Autodesk Inventor part; units mm, degrees
(part 4 of 4)
  line L1289 (-18.1511, -3.5265) -> (-17.9502, -3.8747) construction
  line L1290 (-17.9502, -3.8747) -> (-17.7035, -4.3021) construction
  line L1291 (-17.7035, -4.3021) -> (-17.3591, -4.6088) construction
  line L1292 (-17.3591, -4.6088) -> (-16.8809, -4.76) construction
  line L1293 (-16.8809, -4.76) -> (-16.5137, -4.8761) construction
  line L1294 (-16.5137, -4.8761) -> (-16.1388, -4.8972) construction
  line L1295 (-16.1388, -4.8972) -> (-15.7609, -4.8632) construction
  line L1296 (-15.7609, -4.8632) -> (-15.344, -4.8257) construction
  line L1297 (-15.344, -4.8257) -> (-14.9284, -4.7723) construction
  line L1298 (-14.9284, -4.7723) -> (-14.5126, -4.7225) construction
  line L1299 (-14.5126, -4.7225) -> (-14.3097, -4.6982) construction
  line L1300 (-14.3097, -4.6982) -> (-14.1058, -4.6758) construction
  line L1301 (-14.1058, -4.6758) -> (-13.906, -4.6349) construction
  line L1302 (-13.906, -4.6349) -> (-13.7036, -4.5936) construction
  line L1303 (-13.7036, -4.5936) -> (-13.5886, -4.433) construction
  line L1304 (-13.5886, -4.433) -> (-13.6065, -4.2455) construction
  line L1305 (-13.6065, -4.2455) -> (-13.6174, -4.1315) construction
  line L1306 (-13.6174, -4.1315) -> (-13.6744, -4.0385) construction
  line L1307 (-13.6744, -4.0385) -> (-13.7549, -3.96) construction
  line L1308 (-13.7549, -3.96) -> (-13.9237, -3.7955) construction
  line L1309 (-13.9237, -3.7955) -> (-14.1348, -3.7365) construction
  line L1310 (-14.1348, -3.7365) -> (-14.3597, -3.76) construction
  line L1311 (-14.3597, -3.76) -> (-14.6956, -3.7951) construction
  line L1312 (-14.6956, -3.7951) -> (-15.0291, -3.8532) construction
  line L1313 (-15.0291, -3.8532) -> (-15.364, -3.8988) construction
  line L1314 (-15.364, -3.8988) -> (-15.6048, -3.9316) construction
  line L1315 (-15.6048, -3.9316) -> (-15.8454, -3.9714) construction
  line L1316 (-15.8454, -3.9714) -> (-16.0874, -3.9874) construction
  line L1317 (-16.0874, -3.9874) -> (-16.4238, -4.0097) construction
  line L1318 (-16.4238, -4.0097) -> (-16.7238, -3.9011) construction
  line L1319 (-16.7238, -3.9011) -> (-16.9435, -3.6427) construction
  line L1320 (-16.9435, -3.6427) -> (-17.3408, -3.1754) construction
  line L1321 (-17.3408, -3.1754) -> (-17.5623, -2.6346) construction
  line L1322 (-17.5623, -2.6346) -> (-17.5206, -2.0131) construction
  line L1323 (-17.5206, -2.0131) -> (-17.4887, -1.5389) construction
  line L1324 (-17.4887, -1.5389) -> (-17.2384, -1.2172) construction
  line L1325 (-17.2384, -1.2172) -> (-16.7786, -1.0684) construction
  line L1326 (-16.7786, -1.0684) -> (-16.3846, -0.9409) construction
  line L1327 (-16.3846, -0.9409) -> (-15.9768, -0.89) construction
  line L1328 (-15.9768, -0.89) -> (-15.5673, -0.8506) construction
  line L1329 (-15.5673, -0.8506) -> (-15.3662, -0.8312) construction
  line L1330 (-15.3662, -0.8312) -> (-15.164, -0.8225) construction
  line L1331 (-15.164, -0.8225) -> (-14.9622, -0.8103) construction
  line L1332 (-14.9622, -0.8103) -> (-14.8743, -0.805) construction
  line L1333 (-14.8743, -0.805) -> (-14.7969, -0.7758) construction
  line L1334 (-14.7969, -0.7758) -> (-14.7522, -0.6983) construction
  line L1335 (-14.7522, -0.6983) -> (-14.6073, -0.4469) construction
  line L1336 (-14.6073, -0.4469) -> (-14.6652, -0.192) construction
  line L1337 (-14.6652, -0.192) -> (-14.9177, -0.0574) construction
  line L1338 (-14.9177, -0.0574) -> (-15.0775, 0.0278) construction
  line L1339 (-15.0775, 0.0278) -> (-15.2502, 0.0492) construction
  line L1340 (-15.2502, 0.0492) -> (-15.4261, 0.0563) construction
  line L1341 (-15.4261, 0.0563) -> (-15.7781, 0.0704) construction
  line L1342 (-15.7781, 0.0704) -> (-16.1265, 0.0344) construction
  line L1343 (-16.1265, 0.0344) -> (-16.473, -0.026) construction
  line L1344 (-16.473, -0.026) -> (-16.8039, -0.0836) construction
  line L1345 (-16.8039, -0.0836) -> (-17.133, -0.1458) construction
  line L1346 (-17.133, -0.1458) -> (-17.439, -0.2941) construction
  line L1347 (-17.439, -0.2941) -> (-17.8084, -0.4732) construction
  line L1348 (-17.8084, -0.4732) -> (-18.0982, -0.7312) construction
  line L1349 (-18.0982, -0.7312) -> (-18.265, -1.1138) construction
  line L1350 (-18.265, -1.1138) -> (-18.3824, -1.3828) construction
  line L1351 (-18.3824, -1.3828) -> (-18.4168, -1.6658) construction
  line L1352 (-18.4168, -1.6658) -> (-18.4071, -1.9562) construction
  spline S14 degree 3 poles (-36.9183, 1.2424) (-36.6709, 1.199) (-36.4382, 1.1494) (-36.203, 1.1193) (-35.8877, 1.079) (-35.57, 1.0809) (-35.2581, 1.146) (-35.1542, 1.1676) (-35.0599, 1.235) (-34.9579, 1.283) (-34.9598, 1.2682) (-34.9615, 1.2412) (-34.9669, 1.215) (-35.0299, 0.9055) (-35.0965, 0.5966) (-35.1557, 0.2864) (-35.1823, 0.1473) (-35.1758, 0.1419) (-35.3193, 0.1406) (-35.6164, 0.138) (-35.9136, 0.1414) (-36.2107, 0.1399) (-36.3909, 0.139) (-36.5712, 0.1357) (-36.7512, 0.1286) (-36.8096, 0.1264) (-36.8273, 0.1474) (-36.8315, 0.2021) (-36.855, 0.5079) (-36.8811, 0.8134) (-36.9065, 1.1191) (-36.91, 1.1614) (-36.9146, 1.2037) (-36.9183, 1.2424) knots 0 0 0 0 1 1 1 2 2 2 3 3 3 4 4 4 5 5 5 6 6 6 7 7 7 8 8 8 9 9 9 10 10 10 11 11 11 11
  line L1353 (-36.9183, 1.2424) -> (-36.6709, 1.199) construction
  line L1354 (-36.6709, 1.199) -> (-36.4382, 1.1494) construction
  line L1355 (-36.4382, 1.1494) -> (-36.203, 1.1193) construction
  line L1356 (-36.203, 1.1193) -> (-35.8877, 1.079) construction
  line L1357 (-35.8877, 1.079) -> (-35.57, 1.0809) construction
  line L1358 (-35.57, 1.0809) -> (-35.2581, 1.146) construction
  line L1359 (-35.2581, 1.146) -> (-35.1542, 1.1676) construction
  line L1360 (-35.1542, 1.1676) -> (-35.0599, 1.235) construction
  line L1361 (-35.0599, 1.235) -> (-34.9579, 1.283) construction
  line L1362 (-34.9579, 1.283) -> (-34.9598, 1.2682) construction
  line L1363 (-34.9598, 1.2682) -> (-34.9615, 1.2412) construction
  line L1364 (-34.9615, 1.2412) -> (-34.9669, 1.215) construction
  line L1365 (-34.9669, 1.215) -> (-35.0299, 0.9055) construction
  line L1366 (-35.0299, 0.9055) -> (-35.0965, 0.5966) construction
  line L1367 (-35.0965, 0.5966) -> (-35.1557, 0.2864) construction
  line L1368 (-35.1557, 0.2864) -> (-35.1823, 0.1473) construction
  line L1369 (-35.1823, 0.1473) -> (-35.1758, 0.1419) construction
  line L1370 (-35.1758, 0.1419) -> (-35.3193, 0.1406) construction
  line L1371 (-35.3193, 0.1406) -> (-35.6164, 0.138) construction
  line L1372 (-35.6164, 0.138) -> (-35.9136, 0.1414) construction
  line L1373 (-35.9136, 0.1414) -> (-36.2107, 0.1399) construction
  line L1374 (-36.2107, 0.1399) -> (-36.3909, 0.139) construction
  line L1375 (-36.3909, 0.139) -> (-36.5712, 0.1357) construction
  line L1376 (-36.5712, 0.1357) -> (-36.7512, 0.1286) construction
  line L1377 (-36.7512, 0.1286) -> (-36.8096, 0.1264) construction
  line L1378 (-36.8096, 0.1264) -> (-36.8273, 0.1474) construction
  line L1379 (-36.8273, 0.1474) -> (-36.8315, 0.2021) construction
  line L1380 (-36.8315, 0.2021) -> (-36.855, 0.5079) construction
  line L1381 (-36.855, 0.5079) -> (-36.8811, 0.8134) construction
  line L1382 (-36.8811, 0.8134) -> (-36.9065, 1.1191) construction
  line L1383 (-36.9065, 1.1191) -> (-36.91, 1.1614) construction
  line L1384 (-36.91, 1.1614) -> (-36.9146, 1.2037) construction
  line L1385 (-36.9146, 1.2037) -> (-36.9183, 1.2424) construction
  spline S15 degree 3 poles (-30.21, 0.1155) (-30.4884, 0.1155) (-30.749, 0.1155) (-31.0096, 0.1155) (-31.0949, 0.1155) (-31.1802, 0.1169) (-31.2655, 0.1151) (-31.3106, 0.1141) (-31.3296, 0.129) (-31.3324, 0.1776) (-31.3492, 0.4716) (-31.3731, 0.7652) (-31.386, 1.0594) (-31.3905, 1.1624) (-31.3737, 1.2669) (-31.3602, 1.3699) (-31.3526, 1.4281) (-31.3153, 1.4376) (-31.2641, 1.4089) (-31.105, 1.3198) (-30.9887, 1.1846) (-30.8818, 1.0429) (-30.6662, 0.7573) (-30.4571, 0.4669) (-30.2457, 0.1781) (-30.235, 0.1635) (-30.2276, 0.1466) (-30.21, 0.1155) knots 0 0 0 0 1 1 1 2 2 2 3 3 3 4 4 4 5 5 5 6 6 6 7 7 7 8 8 8 9 9 9 9
  line L1386 (-30.21, 0.1155) -> (-30.4884, 0.1155) construction
  line L1387 (-30.4884, 0.1155) -> (-30.749, 0.1155) construction
  line L1388 (-30.749, 0.1155) -> (-31.0096, 0.1155) construction
  line L1389 (-31.0096, 0.1155) -> (-31.0949, 0.1155) construction
  line L1390 (-31.0949, 0.1155) -> (-31.1802, 0.1169) construction
  line L1391 (-31.1802, 0.1169) -> (-31.2655, 0.1151) construction
  line L1392 (-31.2655, 0.1151) -> (-31.3106, 0.1141) construction
  line L1393 (-31.3106, 0.1141) -> (-31.3296, 0.129) construction
  line L1394 (-31.3296, 0.129) -> (-31.3324, 0.1776) construction
  line L1395 (-31.3324, 0.1776) -> (-31.3492, 0.4716) construction
  line L1396 (-31.3492, 0.4716) -> (-31.3731, 0.7652) construction
  line L1397 (-31.3731, 0.7652) -> (-31.386, 1.0594) construction
  line L1398 (-31.386, 1.0594) -> (-31.3905, 1.1624) construction
  line L1399 (-31.3905, 1.1624) -> (-31.3737, 1.2669) construction
  line L1400 (-31.3737, 1.2669) -> (-31.3602, 1.3699) construction
  line L1401 (-31.3602, 1.3699) -> (-31.3526, 1.4281) construction
  line L1402 (-31.3526, 1.4281) -> (-31.3153, 1.4376) construction
  line L1403 (-31.3153, 1.4376) -> (-31.2641, 1.4089) construction
  line L1404 (-31.2641, 1.4089) -> (-31.105, 1.3198) construction
  line L1405 (-31.105, 1.3198) -> (-30.9887, 1.1846) construction
  line L1406 (-30.9887, 1.1846) -> (-30.8818, 1.0429) construction
  line L1407 (-30.8818, 1.0429) -> (-30.6662, 0.7573) construction
  line L1408 (-30.6662, 0.7573) -> (-30.4571, 0.4669) construction
  line L1409 (-30.4571, 0.4669) -> (-30.2457, 0.1781) construction
  line L1410 (-30.2457, 0.1781) -> (-30.235, 0.1635) construction
  line L1411 (-30.235, 0.1635) -> (-30.2276, 0.1466) construction
  line L1412 (-30.2276, 0.1466) -> (-30.21, 0.1155) construction
  spline S16 degree 3 poles (-33.0561, 0.1374) (-33.4981, 0.1374) (-33.9277, 0.1374) (-34.3711, 0.1374) (-34.3433, 0.2083) (-34.3243, 0.2629) (-34.3009, 0.3155) (-34.2271, 0.4812) (-34.1924, 0.6625) (-34.0848, 0.8154) (-33.9271, 1.0395) (-33.6943, 1.0697) (-33.5072, 0.8689) (-33.4206, 0.7759) (-33.3543, 0.6625) (-33.2866, 0.5536) (-33.2162, 0.4401) (-33.155, 0.3209) (-33.0901, 0.2041) (-33.0787, 0.1836) (-33.0687, 0.1623) (-33.0561, 0.1374) knots 0 0 0 0 1 1 1 2 2 2 3 3 3 4 4 4 5 5 5 6 6 6 7 7 7 7
  line L1413 (-33.0561, 0.1374) -> (-33.4981, 0.1374) construction
  line L1414 (-33.4981, 0.1374) -> (-33.9277, 0.1374) construction
  line L1415 (-33.9277, 0.1374) -> (-34.3711, 0.1374) construction
  line L1416 (-34.3711, 0.1374) -> (-34.3433, 0.2083) construction
  line L1417 (-34.3433, 0.2083) -> (-34.3243, 0.2629) construction
  line L1418 (-34.3243, 0.2629) -> (-34.3009, 0.3155) construction
  line L1419 (-34.3009, 0.3155) -> (-34.2271, 0.4812) construction
  line L1420 (-34.2271, 0.4812) -> (-34.1924, 0.6625) construction
  line L1421 (-34.1924, 0.6625) -> (-34.0848, 0.8154) construction
  line L1422 (-34.0848, 0.8154) -> (-33.9271, 1.0395) construction
  line L1423 (-33.9271, 1.0395) -> (-33.6943, 1.0697) construction
  line L1424 (-33.6943, 1.0697) -> (-33.5072, 0.8689) construction
  line L1425 (-33.5072, 0.8689) -> (-33.4206, 0.7759) construction
  line L1426 (-33.4206, 0.7759) -> (-33.3543, 0.6625) construction
  line L1427 (-33.3543, 0.6625) -> (-33.2866, 0.5536) construction
  line L1428 (-33.2866, 0.5536) -> (-33.2162, 0.4401) construction
  line L1429 (-33.2162, 0.4401) -> (-33.155, 0.3209) construction
  line L1430 (-33.155, 0.3209) -> (-33.0901, 0.2041) construction
  line L1431 (-33.0901, 0.2041) -> (-33.0787, 0.1836) construction
  line L1432 (-33.0787, 0.1836) -> (-33.0687, 0.1623) construction
  line L1433 (-33.0687, 0.1623) -> (-33.0561, 0.1374) construction
  spline S17 degree 3 poles (-36.3665, 2.404) (-36.2371, 2.3846) (-36.0921, 2.3695) (-35.9501, 2.3398) (-35.7931, 2.3069) (-35.7008, 2.1678) (-35.7209, 2.009) (-35.7233, 1.9899) (-35.7495, 1.9609) (-35.767, 1.9589) (-35.9064, 1.9438) (-36.0465, 1.9246) (-36.1863, 1.9252) (-36.351, 1.9258) (-36.5155, 1.9456) (-36.6802, 1.9558) (-36.752, 1.9602) (-36.7965, 1.9968) (-36.8212, 2.0626) (-36.8358, 2.1011) (-36.8552, 2.1379) (-36.8694, 2.1765) (-36.9052, 2.2737) (-36.8786, 2.3317) (-36.7734, 2.3514) (-36.6449, 2.3755) (-36.5139, 2.3856) (-36.3665, 2.404) knots 0 0 0 0 1 1 1 2 2 2 3 3 3 4 4 4 5 5 5 6 6 6 7 7 7 8 8 8 9 9 9 9
  line L1434 (-36.3665, 2.404) -> (-36.2371, 2.3846) construction
  line L1435 (-36.2371, 2.3846) -> (-36.0921, 2.3695) construction
  line L1436 (-36.0921, 2.3695) -> (-35.9501, 2.3398) construction
  line L1437 (-35.9501, 2.3398) -> (-35.7931, 2.3069) construction
  line L1438 (-35.7931, 2.3069) -> (-35.7008, 2.1678) construction
  line L1439 (-35.7008, 2.1678) -> (-35.7209, 2.009) construction
  line L1440 (-35.7209, 2.009) -> (-35.7233, 1.9899) construction
  line L1441 (-35.7233, 1.9899) -> (-35.7495, 1.9609) construction
  line L1442 (-35.7495, 1.9609) -> (-35.767, 1.9589) construction
  line L1443 (-35.767, 1.9589) -> (-35.9064, 1.9438) construction
  line L1444 (-35.9064, 1.9438) -> (-36.0465, 1.9246) construction
  line L1445 (-36.0465, 1.9246) -> (-36.1863, 1.9252) construction
  line L1446 (-36.1863, 1.9252) -> (-36.351, 1.9258) construction
  line L1447 (-36.351, 1.9258) -> (-36.5155, 1.9456) construction
  line L1448 (-36.5155, 1.9456) -> (-36.6802, 1.9558) construction
  line L1449 (-36.6802, 1.9558) -> (-36.752, 1.9602) construction
  line L1450 (-36.752, 1.9602) -> (-36.7965, 1.9968) construction
  line L1451 (-36.7965, 1.9968) -> (-36.8212, 2.0626) construction
  line L1452 (-36.8212, 2.0626) -> (-36.8358, 2.1011) construction
  line L1453 (-36.8358, 2.1011) -> (-36.8552, 2.1379) construction
  line L1454 (-36.8552, 2.1379) -> (-36.8694, 2.1765) construction
  line L1455 (-36.8694, 2.1765) -> (-36.9052, 2.2737) construction
  line L1456 (-36.9052, 2.2737) -> (-36.8786, 2.3317) construction
  line L1457 (-36.8786, 2.3317) -> (-36.7734, 2.3514) construction
  line L1458 (-36.7734, 2.3514) -> (-36.6449, 2.3755) construction
  line L1459 (-36.6449, 2.3755) -> (-36.5139, 2.3856) construction
  line L1460 (-36.5139, 2.3856) -> (-36.3665, 2.404) construction
  spline S18 degree 3 poles (-30.3554, -3.8594) (-30.6123, -3.9168) (-30.8621, -3.9726) (-31.1184, -4.0298) (-31.1033, -3.9732) (-31.0875, -3.9039) (-31.0665, -3.8362) (-31.0168, -3.6764) (-30.9647, -3.5173) (-30.9132, -3.358) (-30.908, -3.3419) (-30.9012, -3.3262) (-30.8937, -3.311) (-30.8561, -3.2345) (-30.8314, -3.2266) (-30.7805, -3.291) (-30.6375, -3.472) (-30.4995, -3.6571) (-30.3601, -3.8409) (-30.3549, -3.8478) (-30.3555, -3.8591) (-30.3554, -3.8594) knots 0 0 0 0 1 1 1 2 2 2 3 3 3 4 4 4 5 5 5 6 6 6 7 7 7 7
  line L1461 (-30.3554, -3.8594) -> (-30.6123, -3.9168) construction
  line L1462 (-30.6123, -3.9168) -> (-30.8621, -3.9726) construction
  line L1463 (-30.8621, -3.9726) -> (-31.1184, -4.0298) construction
  line L1464 (-31.1184, -4.0298) -> (-31.1033, -3.9732) construction
  line L1465 (-31.1033, -3.9732) -> (-31.0875, -3.9039) construction
  line L1466 (-31.0875, -3.9039) -> (-31.0665, -3.8362) construction
  line L1467 (-31.0665, -3.8362) -> (-31.0168, -3.6764) construction
  line L1468 (-31.0168, -3.6764) -> (-30.9647, -3.5173) construction
  line L1469 (-30.9647, -3.5173) -> (-30.9132, -3.358) construction
  line L1470 (-30.9132, -3.358) -> (-30.908, -3.3419) construction
  line L1471 (-30.908, -3.3419) -> (-30.9012, -3.3262) construction
  line L1472 (-30.9012, -3.3262) -> (-30.8937, -3.311) construction
  line L1473 (-30.8937, -3.311) -> (-30.8561, -3.2345) construction
  line L1474 (-30.8561, -3.2345) -> (-30.8314, -3.2266) construction
  line L1475 (-30.8314, -3.2266) -> (-30.7805, -3.291) construction
  line L1476 (-30.7805, -3.291) -> (-30.6375, -3.472) construction
  line L1477 (-30.6375, -3.472) -> (-30.4995, -3.6571) construction
  line L1478 (-30.4995, -3.6571) -> (-30.3601, -3.8409) construction
  line L1479 (-30.3601, -3.8409) -> (-30.3549, -3.8478) construction
  line L1480 (-30.3549, -3.8478) -> (-30.3555, -3.8591) construction
  line L1481 (-30.3555, -3.8591) -> (-30.3554, -3.8594) construction
  spline S19 degree 3 poles (-13.1118, -0.4311) (-12.9758, -0.4017) (-12.8628, -0.3736) (-12.7483, -0.3537) (-12.6473, -0.3362) (-12.578, -0.3894) (-12.5232, -0.4699) (-12.441, -0.5909) (-12.4412, -0.7318) (-12.4222, -0.868) (-12.4138, -0.9278) (-12.4098, -0.9882) (-12.4133, -1.0565) (-12.6633, -0.8759) (-12.8875, -0.6685) (-13.1118, -0.4311) knots 0 0 0 0 1 1 1 2 2 2 3 3 3 4 4 4 5 5 5 5
  line L1482 (-13.1118, -0.4311) -> (-12.9758, -0.4017) construction
  line L1483 (-12.9758, -0.4017) -> (-12.8628, -0.3736) construction
  line L1484 (-12.8628, -0.3736) -> (-12.7483, -0.3537) construction
  line L1485 (-12.7483, -0.3537) -> (-12.6473, -0.3362) construction
  line L1486 (-12.6473, -0.3362) -> (-12.578, -0.3894) construction
  line L1487 (-12.578, -0.3894) -> (-12.5232, -0.4699) construction
  line L1488 (-12.5232, -0.4699) -> (-12.441, -0.5909) construction
  line L1489 (-12.441, -0.5909) -> (-12.4412, -0.7318) construction
  line L1490 (-12.4412, -0.7318) -> (-12.4222, -0.868) construction
  line L1491 (-12.4222, -0.868) -> (-12.4138, -0.9278) construction
  line L1492 (-12.4138, -0.9278) -> (-12.4098, -0.9882) construction
  line L1493 (-12.4098, -0.9882) -> (-12.4133, -1.0565) construction
  line L1494 (-12.4133, -1.0565) -> (-12.6633, -0.8759) construction
  line L1495 (-12.6633, -0.8759) -> (-12.8875, -0.6685) construction
  line L1496 (-12.8875, -0.6685) -> (-13.1118, -0.4311) construction
  spline S20 degree 3 poles (-34.0058, 1.9385) (-33.9591, 2.0472) (-33.9126, 2.1556) (-33.866, 2.2639) (-33.8582, 2.2647) (-33.8504, 2.2656) (-33.8425, 2.2664) (-33.7865, 2.1577) (-33.7306, 2.049) (-33.6737, 1.9385) (-33.7872, 1.9385) (-33.8926, 1.9385) (-34.0058, 1.9385) knots 0 0 0 0 1 1 1 2 2 2 3 3 3 4 4 4 4
  line L1497 (-34.0058, 1.9385) -> (-33.9591, 2.0472) construction
  line L1498 (-33.9591, 2.0472) -> (-33.9126, 2.1556) construction
  line L1499 (-33.9126, 2.1556) -> (-33.866, 2.2639) construction
  line L1500 (-33.866, 2.2639) -> (-33.8582, 2.2647) construction
  line L1501 (-33.8582, 2.2647) -> (-33.8504, 2.2656) construction
  line L1502 (-33.8504, 2.2656) -> (-33.8425, 2.2664) construction
  line L1503 (-33.8425, 2.2664) -> (-33.7865, 2.1577) construction
  line L1504 (-33.7865, 2.1577) -> (-33.7306, 2.049) construction
  line L1505 (-33.7306, 2.049) -> (-33.6737, 1.9385) construction
  line L1506 (-33.6737, 1.9385) -> (-33.7872, 1.9385) construction
  line L1507 (-33.7872, 1.9385) -> (-33.8926, 1.9385) construction
  line L1508 (-33.8926, 1.9385) -> (-34.0058, 1.9385) construction
  spline S21 degree 3 poles (-22.9451, -5.2295) (-22.9442, -4.9431) (-22.8956, -4.6641) (-22.8444, -4.3866) (-22.6649, -3.4153) (-22.3628, -2.4829) (-21.9261, -1.5966) (-21.8333, -1.4082) (-21.7129, -1.231) (-21.5881, -1.0611) (-21.3936, -0.7965) (-21.1315, -0.7284) (-20.8417, -0.8844) (-20.649, -0.9881) (-20.4712, -1.1252) (-20.302, -1.2657) (-19.771, -1.7065) (-19.3209, -2.2247) (-18.8977, -2.7671) (-18.5873, -3.1648) (-18.3021, -3.5799) (-18.055, -4.0201) (-17.9125, -4.2741) (-17.8019, -4.5397) (-17.7696, -4.8335) (-17.7384, -5.1172) (-17.9236, -5.2848) (-18.2033, -5.2157) (-18.4268, -5.1605) (-18.6164, -5.0377) (-18.8006, -4.9046) (-19.1109, -4.6801) (-19.3663, -4.3991) (-19.6171, -4.1137) (-19.7992, -3.9064) (-19.9964, -3.7237) (-20.2668, -3.6352) (-20.612, -3.522) (-20.9998, -3.6362) (-21.2246, -3.9223) (-21.3508, -4.0829) (-21.4456, -4.2596) (-21.5075, -4.4542) (-21.6218, -4.8134) (-21.7813, -5.1515) (-21.9857, -5.4678) (-22.096, -5.6385) (-22.2207, -5.7972) (-22.4026, -5.8994) (-22.6144, -6.0184) (-22.822, -5.9335) (-22.8739, -5.6974) (-22.9076, -5.5437) (-22.922, -5.3856) (-22.9451, -5.2295) knots 0 0 0 0 1 1 1 2 2 2 3 3 3 4 4 4 5 5 5 6 6 6 7 7 7 8 8 8 9 9 9 10 10 10 11 11 11 12 12 12 13 13 13 14 14 14 15 15 15 16 16 16 17 17 17 18 18 18 18
  line L1509 (-22.9451, -5.2295) -> (-22.9442, -4.9431) construction
  line L1510 (-22.9442, -4.9431) -> (-22.8956, -4.6641) construction
  line L1511 (-22.8956, -4.6641) -> (-22.8444, -4.3866) construction
  line L1512 (-22.8444, -4.3866) -> (-22.6649, -3.4153) construction
  line L1513 (-22.6649, -3.4153) -> (-22.3628, -2.4829) construction
  line L1514 (-22.3628, -2.4829) -> (-21.9261, -1.5966) construction
  line L1515 (-21.9261, -1.5966) -> (-21.8333, -1.4082) construction
  line L1516 (-21.8333, -1.4082) -> (-21.7129, -1.231) construction
  line L1517 (-21.7129, -1.231) -> (-21.5881, -1.0611) construction
  line L1518 (-21.5881, -1.0611) -> (-21.3936, -0.7965) construction
  line L1519 (-21.3936, -0.7965) -> (-21.1315, -0.7284) construction
  line L1520 (-21.1315, -0.7284) -> (-20.8417, -0.8844) construction
  line L1521 (-20.8417, -0.8844) -> (-20.649, -0.9881) construction
  line L1522 (-20.649, -0.9881) -> (-20.4712, -1.1252) construction
  line L1523 (-20.4712, -1.1252) -> (-20.302, -1.2657) construction
  line L1524 (-20.302, -1.2657) -> (-19.771, -1.7065) construction
  line L1525 (-19.771, -1.7065) -> (-19.3209, -2.2247) construction
  line L1526 (-19.3209, -2.2247) -> (-18.8977, -2.7671) construction
  line L1527 (-18.8977, -2.7671) -> (-18.5873, -3.1648) construction
  line L1528 (-18.5873, -3.1648) -> (-18.3021, -3.5799) construction
  line L1529 (-18.3021, -3.5799) -> (-18.055, -4.0201) construction
  line L1530 (-18.055, -4.0201) -> (-17.9125, -4.2741) construction
  line L1531 (-17.9125, -4.2741) -> (-17.8019, -4.5397) construction
  line L1532 (-17.8019, -4.5397) -> (-17.7696, -4.8335) construction
  line L1533 (-17.7696, -4.8335) -> (-17.7384, -5.1172) construction
  line L1534 (-17.7384, -5.1172) -> (-17.9236, -5.2848) construction
  line L1535 (-17.9236, -5.2848) -> (-18.2033, -5.2157) construction
  line L1536 (-18.2033, -5.2157) -> (-18.4268, -5.1605) construction
  line L1537 (-18.4268, -5.1605) -> (-18.6164, -5.0377) construction
  line L1538 (-18.6164, -5.0377) -> (-18.8006, -4.9046) construction
  line L1539 (-18.8006, -4.9046) -> (-19.1109, -4.6801) construction
  line L1540 (-19.1109, -4.6801) -> (-19.3663, -4.3991) construction
  line L1541 (-19.3663, -4.3991) -> (-19.6171, -4.1137) construction
  line L1542 (-19.6171, -4.1137) -> (-19.7992, -3.9064) construction
  line L1543 (-19.7992, -3.9064) -> (-19.9964, -3.7237) construction
  line L1544 (-19.9964, -3.7237) -> (-20.2668, -3.6352) construction
  line L1545 (-20.2668, -3.6352) -> (-20.612, -3.522) construction
  line L1546 (-20.612, -3.522) -> (-20.9998, -3.6362) construction
  line L1547 (-20.9998, -3.6362) -> (-21.2246, -3.9223) construction
  line L1548 (-21.2246, -3.9223) -> (-21.3508, -4.0829) construction
  line L1549 (-21.3508, -4.0829) -> (-21.4456, -4.2596) construction
  line L1550 (-21.4456, -4.2596) -> (-21.5075, -4.4542) construction
  line L1551 (-21.5075, -4.4542) -> (-21.6218, -4.8134) construction
  line L1552 (-21.6218, -4.8134) -> (-21.7813, -5.1515) construction
  line L1553 (-21.7813, -5.1515) -> (-21.9857, -5.4678) construction
  line L1554 (-21.9857, -5.4678) -> (-22.096, -5.6385) construction
  line L1555 (-22.096, -5.6385) -> (-22.2207, -5.7972) construction
  line L1556 (-22.2207, -5.7972) -> (-22.4026, -5.8994) construction
  line L1557 (-22.4026, -5.8994) -> (-22.6144, -6.0184) construction
  line L1558 (-22.6144, -6.0184) -> (-22.822, -5.9335) construction
  line L1559 (-22.822, -5.9335) -> (-22.8739, -5.6974) construction
  line L1560 (-22.8739, -5.6974) -> (-22.9076, -5.5437) construction
  line L1561 (-22.9076, -5.5437) -> (-22.922, -5.3856) construction
  line L1562 (-22.922, -5.3856) -> (-22.9451, -5.2295) construction
  spline S22 degree 3 poles (-21.0271, -1.7855) (-21.1843, -2.0357) (-21.2431, -2.3095) (-21.301, -2.5729) (-21.0442, -2.5176) (-20.7906, -2.463) (-20.5321, -2.4074) (-20.6938, -2.2008) (-20.8254, -1.9696) (-21.0271, -1.7855) knots 0 0 0 0 1 1 1 2 2 2 3 3 3 3
  line L1563 (-21.0271, -1.7855) -> (-21.1843, -2.0357) construction
  line L1564 (-21.1843, -2.0357) -> (-21.2431, -2.3095) construction
  line L1565 (-21.2431, -2.3095) -> (-21.301, -2.5729) construction
  line L1566 (-21.301, -2.5729) -> (-21.0442, -2.5176) construction
  line L1567 (-21.0442, -2.5176) -> (-20.7906, -2.463) construction
  line L1568 (-20.7906, -2.463) -> (-20.5321, -2.4074) construction
  line L1569 (-20.5321, -2.4074) -> (-20.6938, -2.2008) construction
  line L1570 (-20.6938, -2.2008) -> (-20.8254, -1.9696) construction
  line L1571 (-20.8254, -1.9696) -> (-21.0271, -1.7855) construction
  spline S23 degree 3 poles (-18.4071, -1.9562) (-18.4168, -1.6658) (-18.3824, -1.3828) (-18.265, -1.1138) (-18.0982, -0.7312) (-17.8084, -0.4732) (-17.439, -0.2941) (-17.133, -0.1458) (-16.8039, -0.0836) (-16.473, -0.026) (-16.1265, 0.0344) (-15.7781, 0.0704) (-15.4261, 0.0563) (-15.2502, 0.0492) (-15.0775, 0.0278) (-14.9177, -0.0574) (-14.6652, -0.192) (-14.6073, -0.4469) (-14.7522, -0.6983) (-14.7969, -0.7758) (-14.8743, -0.805) (-14.9622, -0.8103) (-15.164, -0.8225) (-15.3662, -0.8312) (-15.5673, -0.8506) (-15.9768, -0.89) (-16.3846, -0.9409) (-16.7786, -1.0684) (-17.2384, -1.2172) (-17.4887, -1.5389) (-17.5206, -2.0131) (-17.5623, -2.6346) (-17.3408, -3.1754) (-16.9435, -3.6427) (-16.7238, -3.9011) (-16.4238, -4.0097) (-16.0874, -3.9874) (-15.8454, -3.9714) (-15.6048, -3.9316) (-15.364, -3.8988) (-15.0291, -3.8532) (-14.6956, -3.7951) (-14.3597, -3.76) (-14.1348, -3.7365) (-13.9237, -3.7955) (-13.7549, -3.96) (-13.6744, -4.0385) (-13.6174, -4.1315) (-13.6065, -4.2455) (-13.5886, -4.433) (-13.7036, -4.5936) (-13.906, -4.6349) (-14.1058, -4.6758) (-14.3097, -4.6982) (-14.5126, -4.7225) (-14.9284, -4.7723) (-15.344, -4.8257) (-15.7609, -4.8632) (-16.1388, -4.8972) (-16.5137, -4.8761) (-16.8809, -4.76) (-17.3591, -4.6088) (-17.7035, -4.3021) (-17.9502, -3.8747) (-18.1511, -3.5265) (-18.2602, -3.146) (-18.3273, -2.7539) (-18.3722, -2.4908) (-18.3953, -2.224) (-18.4281, -1.9589) (-18.4211, -1.958) (-18.4141, -1.9571) (-18.4071, -1.9562) knots 0 0 0 0 1 1 1 2 2 2 3 3 3 4 4 4 5 5 5 6 6 6 7 7 7 8 8 8 9 9 9 10 10 10 11 11 11 12 12 12 13 13 13 14 14 14 15 15 15 16 16 16 17 17 17 18 18 18 19 19 19 20 20 20 21 21 21 22 22 22 23 23 23 24 24 24 24
  line L1572 (-18.4071, -1.9562) -> (-18.4168, -1.6658) construction
  line L1573 (-18.4168, -1.6658) -> (-18.3824, -1.3828) construction
  line L1574 (-18.3824, -1.3828) -> (-18.265, -1.1138) construction
  line L1575 (-18.265, -1.1138) -> (-18.0982, -0.7312) construction
  line L1576 (-18.0982, -0.7312) -> (-17.8084, -0.4732) construction
  line L1577 (-17.8084, -0.4732) -> (-17.439, -0.2941) construction
  line L1578 (-17.439, -0.2941) -> (-17.133, -0.1458) construction
  line L1579 (-17.133, -0.1458) -> (-16.8039, -0.0836) construction
  line L1580 (-16.8039, -0.0836) -> (-16.473, -0.026) construction
  line L1581 (-16.473, -0.026) -> (-16.1265, 0.0344) construction
  line L1582 (-16.1265, 0.0344) -> (-15.7781, 0.0704) construction
  line L1583 (-15.7781, 0.0704) -> (-15.4261, 0.0563) construction
  line L1584 (-15.4261, 0.0563) -> (-15.2502, 0.0492) construction
  line L1585 (-15.2502, 0.0492) -> (-15.0775, 0.0278) construction
  line L1586 (-15.0775, 0.0278) -> (-14.9177, -0.0574) construction
  line L1587 (-14.9177, -0.0574) -> (-14.6652, -0.192) construction
  line L1588 (-14.6652, -0.192) -> (-14.6073, -0.4469) construction
  line L1589 (-14.6073, -0.4469) -> (-14.7522, -0.6983) construction
  line L1590 (-14.7522, -0.6983) -> (-14.7969, -0.7758) construction
  line L1591 (-14.7969, -0.7758) -> (-14.8743, -0.805) construction
  line L1592 (-14.8743, -0.805) -> (-14.9622, -0.8103) construction
  line L1593 (-14.9622, -0.8103) -> (-15.164, -0.8225) construction
  line L1594 (-15.164, -0.8225) -> (-15.3662, -0.8312) construction
  line L1595 (-15.3662, -0.8312) -> (-15.5673, -0.8506) construction
  line L1596 (-15.5673, -0.8506) -> (-15.9768, -0.89) construction
  line L1597 (-15.9768, -0.89) -> (-16.3846, -0.9409) construction
  line L1598 (-16.3846, -0.9409) -> (-16.7786, -1.0684) construction
  line L1599 (-16.7786, -1.0684) -> (-17.2384, -1.2172) construction
  line L1600 (-17.2384, -1.2172) -> (-17.4887, -1.5389) construction
  line L1601 (-17.4887, -1.5389) -> (-17.5206, -2.0131) construction
  line L1602 (-17.5206, -2.0131) -> (-17.5623, -2.6346) construction
  line L1603 (-17.5623, -2.6346) -> (-17.3408, -3.1754) construction
  line L1604 (-17.3408, -3.1754) -> (-16.9435, -3.6427) construction
  line L1605 (-16.9435, -3.6427) -> (-16.7238, -3.9011) construction
  line L1606 (-16.7238, -3.9011) -> (-16.4238, -4.0097) construction
  line L1607 (-16.4238, -4.0097) -> (-16.0874, -3.9874) construction
  line L1608 (-16.0874, -3.9874) -> (-15.8454, -3.9714) construction
  line L1609 (-15.8454, -3.9714) -> (-15.6048, -3.9316) construction
  line L1610 (-15.6048, -3.9316) -> (-15.364, -3.8988) construction
  line L1611 (-15.364, -3.8988) -> (-15.0291, -3.8532) construction
  line L1612 (-15.0291, -3.8532) -> (-14.6956, -3.7951) construction
  line L1613 (-14.6956, -3.7951) -> (-14.3597, -3.76) construction
  line L1614 (-14.3597, -3.76) -> (-14.1348, -3.7365) construction
  line L1615 (-14.1348, -3.7365) -> (-13.9237, -3.7955) construction
  line L1616 (-13.9237, -3.7955) -> (-13.7549, -3.96) construction
  line L1617 (-13.7549, -3.96) -> (-13.6744, -4.0385) construction
  line L1618 (-13.6744, -4.0385) -> (-13.6174, -4.1315) construction
  line L1619 (-13.6174, -4.1315) -> (-13.6065, -4.2455) construction
  line L1620 (-13.6065, -4.2455) -> (-13.5886, -4.433) construction
  line L1621 (-13.5886, -4.433) -> (-13.7036, -4.5936) construction
  line L1622 (-13.7036, -4.5936) -> (-13.906, -4.6349) construction
  line L1623 (-13.906, -4.6349) -> (-14.1058, -4.6758) construction
  line L1624 (-14.1058, -4.6758) -> (-14.3097, -4.6982) construction
  line L1625 (-14.3097, -4.6982) -> (-14.5126, -4.7225) construction
  line L1626 (-14.5126, -4.7225) -> (-14.9284, -4.7723) construction
  line L1627 (-14.9284, -4.7723) -> (-15.344, -4.8257) construction
  line L1628 (-15.344, -4.8257) -> (-15.7609, -4.8632) construction
  line L1629 (-15.7609, -4.8632) -> (-16.1388, -4.8972) construction
  line L1630 (-16.1388, -4.8972) -> (-16.5137, -4.8761) construction
  line L1631 (-16.5137, -4.8761) -> (-16.8809, -4.76) construction
  line L1632 (-16.8809, -4.76) -> (-17.3591, -4.6088) construction
  line L1633 (-17.3591, -4.6088) -> (-17.7035, -4.3021) construction
  line L1634 (-17.7035, -4.3021) -> (-17.9502, -3.8747) construction
  line L1635 (-17.9502, -3.8747) -> (-18.1511, -3.5265) construction
  line L1636 (-18.1511, -3.5265) -> (-18.2602, -3.146) construction
  line L1637 (-18.2602, -3.146) -> (-18.3273, -2.7539) construction
  line L1638 (-18.3273, -2.7539) -> (-18.3722, -2.4908) construction
  line L1639 (-18.3722, -2.4908) -> (-18.3953, -2.224) construction
  line L1640 (-18.3953, -2.224) -> (-18.4281, -1.9589) construction
  line L1641 (-18.4281, -1.9589) -> (-18.4211, -1.958) construction
  line L1642 (-18.4211, -1.958) -> (-18.4141, -1.9571) construction
  line L1643 (-18.4141, -1.9571) -> (-18.4071, -1.9562) construction
  spline S24 degree 3 poles (-21.0271, -1.7855) (-20.8254, -1.9696) (-20.6938, -2.2008) (-20.5321, -2.4074) (-20.7906, -2.463) (-21.0442, -2.5176) (-21.301, -2.5729) (-21.2431, -2.3095) (-21.1843, -2.0357) (-21.0271, -1.7855) knots 0 0 0 0 1 1 1 2 2 2 3 3 3 3
  line L1644 (-21.0271, -1.7855) -> (-20.8254, -1.9696) construction
  line L1645 (-20.8254, -1.9696) -> (-20.6938, -2.2008) construction
  line L1646 (-20.6938, -2.2008) -> (-20.5321, -2.4074) construction
  line L1647 (-20.5321, -2.4074) -> (-20.7906, -2.463) construction
  line L1648 (-20.7906, -2.463) -> (-21.0442, -2.5176) construction
  line L1649 (-21.0442, -2.5176) -> (-21.301, -2.5729) construction
  line L1650 (-21.301, -2.5729) -> (-21.2431, -2.3095) construction
  line L1651 (-21.2431, -2.3095) -> (-21.1843, -2.0357) construction
  line L1652 (-21.1843, -2.0357) -> (-21.0271, -1.7855) construction
  point P0 (0, 0)
  constraints: 41 other
extrude "Extrusion30" cut sketch "Sketch31" against normal blind 1 bodies 15
sketch "Sketch32" plane through (19.3, 13.025, 8.1) normal (0, 0, 1) x (1, 0, 0)
  line L0 (-23.4743, -26.7226) -> (5.6725, -26.7226) construction
  line L1 (5.6725, -26.7226) -> (5.6725, -29.7726) construction
  line L2 (5.6725, -29.7726) -> (-23.4743, -29.7726) construction
  line L3 (-23.4743, -29.7726) -> (-23.4743, -26.7226) construction
  line L4 (-23.1859, -29.2626) -> (-23.1859, -26.7226)
  line L5 (-23.1859, -26.7226) -> (-20.8397, -26.7226)
  line L6 (-20.8397, -26.7226) -> (-20.8397, -27.0494)
  line L7 (-20.8397, -27.0494) -> (-22.6472, -27.0494)
  line L8 (-22.6472, -27.0494) -> (-22.6472, -27.7414)
  line L9 (-22.6472, -27.7414) -> (-21.0313, -27.7414)
  line L10 (-21.0313, -27.7414) -> (-21.0313, -28.0681)
  line L11 (-21.0313, -28.0681) -> (-22.6472, -28.0681)
  line L12 (-22.6472, -28.0681) -> (-22.6472, -28.9358)
  line L13 (-22.6472, -28.9358) -> (-20.8397, -28.9358)
  line L14 (-20.8397, -28.9358) -> (-20.8397, -29.2626)
  line L15 (-20.8397, -29.2626) -> (-23.1859, -29.2626)
  line L16 (-20.3777, -29.2626) -> (-20.3777, -28.9358)
  line L17 (-20.3777, -28.9358) -> (-18.6468, -28.9358)
  spline S0 degree 2 poles (-18.6468, -28.9358) (-18.4935, -28.9358) (-18.4935, -28.8119) knots 0 0 0 1 1 1
  line L18 (-18.4935, -28.8119) -> (-18.4935, -28.1921)
  spline S1 degree 2 poles (-18.4935, -28.1921) (-18.4935, -28.0681) (-18.6468, -28.0681) knots 0 0 0 1 1 1
  line L19 (-18.6468, -28.0681) -> (-19.8007, -28.0681)
  spline S2 degree 2 poles (-19.8007, -28.0681) (-20.3777, -28.0681) (-20.3777, -27.6061) knots 0 0 0 1 1 1
  line L20 (-20.3777, -27.6061) -> (-20.3777, -27.1847)
  spline S3 degree 2 poles (-20.3777, -27.1847) (-20.3777, -26.7226) (-19.8007, -26.7226) knots 0 0 0 1 1 1
  line L21 (-19.8007, -26.7226) -> (-18.1464, -26.7226)
  line L22 (-18.1464, -26.7226) -> (-18.1464, -27.0494)
  line L23 (-18.1464, -27.0494) -> (-19.6858, -27.0494)
  spline S4 degree 2 poles (-19.6858, -27.0494) (-19.839, -27.0494) (-19.839, -27.1734) knots 0 0 0 1 1 1
  line L24 (-19.839, -27.1734) -> (-19.839, -27.6174)
  spline S5 degree 2 poles (-19.839, -27.6174) (-19.839, -27.7414) (-19.6858, -27.7414) knots 0 0 0 1 1 1
  line L25 (-19.6858, -27.7414) -> (-18.5318, -27.7414)
  spline S6 degree 2 poles (-18.5318, -27.7414) (-17.9549, -27.7414) (-17.9549, -28.2034) knots 0 0 0 1 1 1
  line L26 (-17.9549, -28.2034) -> (-17.9549, -28.8006)
  spline S7 degree 2 poles (-17.9549, -28.8006) (-17.9549, -29.2626) (-18.5318, -29.2626) knots 0 0 0 1 1 1
  line L27 (-18.5318, -29.2626) -> (-20.3777, -29.2626)
  line L28 (-17.4162, -29.2626) -> (-17.4162, -26.7226)
  line L29 (-17.4162, -26.7226) -> (-15.5704, -26.7226)
  spline S8 degree 2 poles (-15.5704, -26.7226) (-14.9934, -26.7226) (-14.9934, -27.1847) knots 0 0 0 1 1 1
  line L30 (-14.9934, -27.1847) -> (-14.9934, -27.7999)
  spline S9 degree 2 poles (-14.9934, -27.7999) (-14.9934, -28.262) (-15.5704, -28.262) knots 0 0 0 1 1 1
  line L31 (-15.5704, -28.262) -> (-16.8776, -28.262)
  line L32 (-16.8776, -28.262) -> (-16.8776, -29.2626)
  line L33 (-16.8776, -29.2626) -> (-17.4162, -29.2626)
  line L34 (-16.8776, -27.9352) -> (-15.6853, -27.9352)
  spline S10 degree 2 poles (-15.6853, -27.9352) (-15.5321, -27.9352) (-15.5321, -27.8112) knots 0 0 0 1 1 1
  line L35 (-15.5321, -27.8112) -> (-15.5321, -27.1734)
  spline S11 degree 2 poles (-15.5321, -27.1734) (-15.5321, -27.0494) (-15.6853, -27.0494) knots 0 0 0 1 1 1
  line L36 (-15.6853, -27.0494) -> (-16.8776, -27.0494)
  line L37 (-16.8776, -27.0494) -> (-16.8776, -27.9352)
  line L38 (-14.4728, -29.2626) -> (-14.4728, -28.9358)
  line L39 (-14.4728, -28.9358) -> (-12.9718, -28.9358)
  spline S12 degree 2 poles (-12.9718, -28.9358) (-12.8185, -28.9358) (-12.8185, -28.8119) knots 0 0 0 1 1 1
  line L40 (-12.8185, -28.8119) -> (-12.8185, -28.1921)
  spline S13 degree 2 poles (-12.8185, -28.1921) (-12.8185, -28.0681) (-12.9718, -28.0681) knots 0 0 0 1 1 1
  line L41 (-12.9718, -28.0681) -> (-14.1257, -28.0681)
  line L42 (-14.1257, -28.0681) -> (-14.1257, -27.7414)
  line L43 (-14.1257, -27.7414) -> (-12.9718, -27.7414)
  spline S14 degree 2 poles (-12.9718, -27.7414) (-12.8185, -27.7414) (-12.8185, -27.6174) knots 0 0 0 1 1 1
  line L44 (-12.8185, -27.6174) -> (-12.8185, -27.1734)
  spline S15 degree 2 poles (-12.8185, -27.1734) (-12.8185, -27.0494) (-12.9718, -27.0494) knots 0 0 0 1 1 1
  line L45 (-12.9718, -27.0494) -> (-14.4728, -27.0494)
  line L46 (-14.4728, -27.0494) -> (-14.4728, -26.7226)
  line L47 (-14.4728, -26.7226) -> (-12.8568, -26.7226)
  spline S16 degree 2 poles (-12.8568, -26.7226) (-12.2799, -26.7226) (-12.2799, -27.1847) knots 0 0 0 1 1 1
  line L48 (-12.2799, -27.1847) -> (-12.2799, -27.4799)
  spline S17 degree 2 poles (-12.2799, -27.4799) (-12.2799, -27.7954) (-12.5481, -27.8946) knots 0 0 0 1 1 1
  spline S18 degree 2 poles (-12.5481, -27.8946) (-12.2799, -27.996) (-12.2799, -28.3116) knots 0 0 0 1 1 1
  line L49 (-12.2799, -28.3116) -> (-12.2799, -28.8006)
  spline S19 degree 2 poles (-12.2799, -28.8006) (-12.2799, -29.2626) (-12.8568, -29.2626) knots 0 0 0 1 1 1
  line L50 (-12.8568, -29.2626) -> (-14.4728, -29.2626)
  line L51 (-11.8201, -29.2626) -> (-11.8201, -28.2034)
  spline S20 degree 2 poles (-11.8201, -28.2034) (-11.8201, -27.7414) (-11.2431, -27.7414) knots 0 0 0 1 1 1
  line L52 (-11.2431, -27.7414) -> (-10.2425, -27.7414)
  spline S21 degree 2 poles (-10.2425, -27.7414) (-10.0892, -27.7414) (-10.0892, -27.6174) knots 0 0 0 1 1 1
  line L53 (-10.0892, -27.6174) -> (-10.0892, -27.1734)
  spline S22 degree 2 poles (-10.0892, -27.1734) (-10.0892, -27.0494) (-10.2425, -27.0494) knots 0 0 0 1 1 1
  line L54 (-10.2425, -27.0494) -> (-11.6285, -27.0494)
  line L55 (-11.6285, -27.0494) -> (-11.6285, -26.7226)
  line L56 (-11.6285, -26.7226) -> (-10.1275, -26.7226)
  spline S23 degree 2 poles (-10.1275, -26.7226) (-9.5506, -26.7226) (-9.5506, -27.1847) knots 0 0 0 1 1 1
  line L57 (-9.5506, -27.1847) -> (-9.5506, -27.6061)
  spline S24 degree 2 poles (-9.5506, -27.6061) (-9.5506, -28.0681) (-10.1275, -28.0681) knots 0 0 0 1 1 1
  line L58 (-10.1275, -28.0681) -> (-11.1282, -28.0681)
  spline S25 degree 2 poles (-11.1282, -28.0681) (-11.2814, -28.0681) (-11.2814, -28.1921) knots 0 0 0 1 1 1
  line L59 (-11.2814, -28.1921) -> (-11.2814, -28.9358)
  line L60 (-11.2814, -28.9358) -> (-9.5506, -28.9358)
  line L61 (-9.5506, -28.9358) -> (-9.5506, -29.2626)
  line L62 (-9.5506, -29.2626) -> (-11.8201, -29.2626)
  line L63 (-7.7994, -28.8006) -> (-7.7994, -27.1847)
  spline S26 degree 2 poles (-7.7994, -27.1847) (-7.7994, -26.7226) (-7.2224, -26.7226) knots 0 0 0 1 1 1
  line L64 (-7.2224, -26.7226) -> (-5.4532, -26.7226)
  line L65 (-5.4532, -26.7226) -> (-5.4532, -27.0494)
  line L66 (-5.4532, -27.0494) -> (-7.1075, -27.0494)
  spline S27 degree 2 poles (-7.1075, -27.0494) (-7.2607, -27.0494) (-7.2607, -27.1734) knots 0 0 0 1 1 1
  line L67 (-7.2607, -27.1734) -> (-7.2607, -28.8119)
  spline S28 degree 2 poles (-7.2607, -28.8119) (-7.2607, -28.9358) (-7.1075, -28.9358) knots 0 0 0 1 1 1
  line L68 (-7.1075, -28.9358) -> (-5.4532, -28.9358)
  line L69 (-5.4532, -28.9358) -> (-5.4532, -29.2626)
  line L70 (-5.4532, -29.2626) -> (-7.2224, -29.2626)
  spline S29 degree 2 poles (-7.2224, -29.2626) (-7.7994, -29.2626) (-7.7994, -28.8006) knots 0 0 0 1 1 1
  line L71 (-5.0295, -28.8322) -> (-5.0295, -28.5775)
  spline S30 degree 2 poles (-5.0295, -28.5775) (-5.0295, -28.147) (-4.4908, -28.147) knots 0 0 0 1 1 1
  line L72 (-4.4908, -28.147) -> (-3.5668, -28.147)
  line L73 (-3.5668, -28.147) -> (-3.5668, -27.8135)
  spline S31 degree 2 poles (-3.5668, -27.8135) (-3.5668, -27.7053) (-3.702, -27.7053) knots 0 0 0 1 1 1
  line L74 (-3.702, -27.7053) -> (-4.8762, -27.7053)
  line L75 (-4.8762, -27.7053) -> (-4.8762, -27.4168)
  line L76 (-4.8762, -27.4168) -> (-3.6051, -27.4168)
  spline S32 degree 2 poles (-3.6051, -27.4168) (-3.0665, -27.4168) (-3.0665, -27.8473) knots 0 0 0 1 1 1
  line L77 (-3.0665, -27.8473) -> (-3.0665, -29.2626)
  line L78 (-3.0665, -29.2626) -> (-4.4908, -29.2626)
  spline S33 degree 2 poles (-4.4908, -29.2626) (-5.0295, -29.2626) (-5.0295, -28.8322) knots 0 0 0 1 1 1
  spline S34 degree 2 poles (-4.5291, -28.866) (-4.5291, -28.9742) (-4.3939, -28.9742) knots 0 0 0 1 1 1
  line L79 (-4.3939, -28.9742) -> (-3.5668, -28.9742)
  line L80 (-3.5668, -28.9742) -> (-3.5668, -28.4355)
  line L81 (-3.5668, -28.4355) -> (-4.3939, -28.4355)
  spline S35 degree 2 poles (-4.3939, -28.4355) (-4.5291, -28.4355) (-4.5291, -28.5437) knots 0 0 0 1 1 1
  line L82 (-4.5291, -28.5437) -> (-4.5291, -28.866)
  line L83 (-2.5661, -29.2626) -> (-2.5661, -27.4168)
  line L84 (-2.5661, -27.4168) -> (0.0099, -27.4168)
  spline S36 degree 2 poles (0.0099, -27.4168) (0.5486, -27.4168) (0.5486, -27.8473) knots 0 0 0 1 1 1
  line L85 (0.5486, -27.8473) -> (0.5486, -29.2626)
  line L86 (0.5486, -29.2626) -> (0.0483, -29.2626)
  line L87 (0.0483, -29.2626) -> (0.0483, -27.8135)
  spline S37 degree 2 poles (0.0483, -27.8135) (0.0483, -27.7053) (-0.087, -27.7053) knots 0 0 0 1 1 1
  line L88 (-0.087, -27.7053) -> (-0.7586, -27.7053)
  line L89 (-0.7586, -27.7053) -> (-0.7586, -29.2626)
  line L90 (-0.7586, -29.2626) -> (-1.2589, -29.2626)
  line L91 (-1.2589, -29.2626) -> (-1.2589, -27.8135)
  spline S38 degree 2 poles (-1.2589, -27.8135) (-1.2589, -27.7053) (-1.3942, -27.7053) knots 0 0 0 1 1 1
  line L92 (-1.3942, -27.7053) -> (-2.0658, -27.7053)
  line L93 (-2.0658, -27.7053) -> (-2.0658, -29.2626)
  line L94 (-2.0658, -29.2626) -> (-2.5661, -29.2626)
  point P0 (-19.3, -13.025)
  constraints: 2 other
extrude "Extrusion31" cut sketch "Sketch32" against normal blind 1 bodies 15
equation "\"d2\" = 0.5 * d1"
equation "\"d3\" = 0.5 * d0"
equation "\"d20\" = 0.5 * d19"
equation "\"d21\" = 0.5 * d22"
equation "\"d54\" = d53"
equation "\"d69\" = 0.5 * d70"
equation "\"d71\" = 0.5 * d72"
equation "\"d97\" = d96"
equation "\"d99\" = d98"
equation "\"d100\" = d99"
equation "\"d101\" = d99"
equation "\"d102\" = d98"
equation "\"d149\" = d148"
equation "\"d150\" = d148"
equation "\"d151\" = d148"
equation "\"d189\" = d185"
equation "\"d242\" = d241"
equation "\"d96\" = 0.85"
body "Solid1"
body "Solid2"
body "Solid3"
body "Solid4"
body "Solid5"
body "Solid6"
body "Solid7"
body "Solid8"
body "Solid9"
body "Solid10"
body "Solid11"
body "Solid12"
body "Solid13"
body "Solid14"
